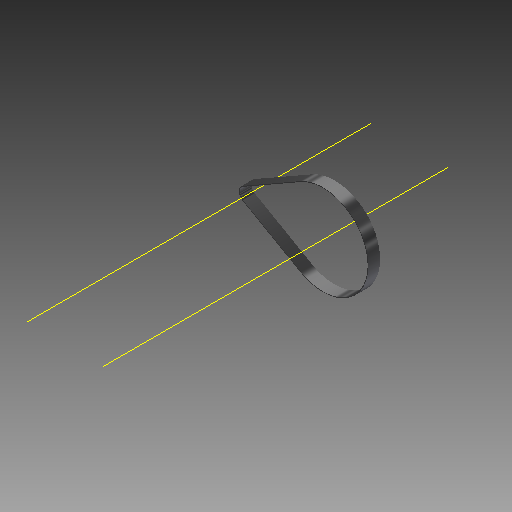
# Autodesk Inventor part: Synchronous Belt
Saved by Autodesk Inventor 2017 (Build 210142000, 142)
## iProperties
Created: 2018-04-16
Part Number: Synchronous Belt
Material: Rubber
Document SubType Name: Modeling
Designer: RKL
Density: 1 g/cm^3
Appearance: Rubber - Black - Version 1.1
CustomPartVersion: 1
Author: RKL
Autodesk Inventor part; units mm, degrees
sketch "Sketch Path" plane through (0, 0, 0) normal (0, 0, 1) x (1, 0, 0)
  arc A0 (-102.9615, 5.1817) -> (-102.9615, -5.1817) centre (-100, 0) ccw
  arc A1 (-54.0022, -33.1631) -> (-54.0022, 33.1631) centre (-35.0487, 0) ccw
  line L0 (-54.0022, -33.1631) -> (-102.9615, -5.1817)
  line L1 (-102.9615, 5.1817) -> (-54.0022, 33.1631)
  constraints: 4 end point, 4 point on circle, 2 centre point
ref_plane "Cross Section Plane" through (-102.9615, -5.1817, 0) normal (0.8682, -0.4962, 0) x (0, 0, 1)
ref_plane "Work Plane2" through (-100, 0, 0) normal (-1, 0, 0) x (0, 0, 1)
ref_plane "Work Plane3" through (-35.0487, 0, 0) normal (-0.8895, -0.4569, 0) x (0, 0, 1)
sketch "Cross Section" plane through (-102.9615, -5.1817, 0) normal (0.8682, -0.4962, 0) x (0, 0, 1)
  line L0 (-5, 0.3) -> (5, 0.3)
  line L1 (5, 0.3) -> (5, -0.3)
  line L2 (5, -0.3) -> (-5, -0.3)
  line L3 (-5, -0.3) -> (-5, 0.3)
  line L4 (-5, 0) -> (5, 0) construction
  point P0 (0, 0)
  point P1 (0, 0)
  dimension "d0" = 10
  dimension "d4" = 0.3
  dimension "d5" = 0.3
  constraints: 10 end point, 3 midpoint, 2 parallel, 1 coincident, 1 horizontal, 1 perpendicular, 1 other
  measures "d0" distance between parallel lines of L1 L3
  measures "d4" distance between parallel lines of L2 L4
  measures "d5" distance between parallel lines of L4 L0
sweep "Belt" add profiles "Cross Section" path "Sketch Path"
equation "\"d0\" = da_B"
equation "\"d4\" = da_a"
equation "\"d5\" = da_a2"
equation "\"da_B\" = 10"
equation "\"da_pb\" = 2.5"
equation "\"da_L\" = 285"
equation "\"da_a\" = 0.3"
equation "\"da_S\" = 1.5"
equation "\"da_Beta\" = 20deg"
equation "\"da_Ht\" = 0.7"
equation "\"da_H\" = 1.3"
equation "\"da_a2\" = 0.3"
body "Solid1"
